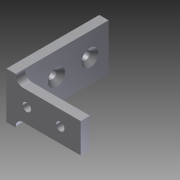
# Autodesk Inventor part: 13_0204_014
Saved by Autodesk Inventor 2012 SP1 (Build 160190100, 190)
## iProperties
Created: 2013-03-28
Part Number: 13_0204_014
Material: Default
Document SubType Name: Modeling
Designer: vogel
Density: 1 g/cm^3
Author: vogel
Autodesk Inventor part; units mm, degrees
ref_plane "YZ Plane" through (0, 0, 0) normal (1, 0, 0) x (0, 1, 0)
ref_plane "XZ Plane" through (0, 0, 0) normal (0, 1, 0) x (-1, 0, 0)
ref_plane "XY Plane" through (0, 0, 0) normal (0, 0, 1) x (1, 0, 0)
sketch "Skizze1" plane through (0, 0, 0) normal (0, 0, 1) x (1, 0, 0)
  line L0 (5, 5) -> (5, 50)
  line L1 (5, 50) -> (0, 50)
  line L2 (0, 50) -> (0, 0)
  line L3 (5, 5) -> (50, 5)
  line L4 (50, 5) -> (50, 0)
  line L5 (-10, 0) -> (60, 0) projected
  line L6 (0, -10) -> (0, 60) projected
  line L7 (0, 0) -> (50, 0)
  dimension "d3" = 5
  dimension "d4" = 5
  dimension "d5" = 50
  dimension "d6" = 50
  constraints: 12 end point, 2 collinear, 2 perpendicular, 1 horizontal, 1 parallel
  measures "d3" distance between parallel lines of L0 L2
  measures "d4" distance between parallel lines of L5 L3
  measures "d5" distance of L1.end L2.end
  measures "d6" distance of L2.end L4.end
extrude "Extrusion1" add sketch "Skizze1" along normal blind 25
sketch "Skizze3" plane through (0, 0, 0) normal (0, -1, 0) x (1, 0, 0)
  line L0 (0, 0) -> (0, 25) projected
  line L1 (50, 0) -> (0, 0) projected
  line L2 (50, 0) -> (50, 25) projected
  line L3 (50, 25) -> (40, 25)
  line L4 (40, 25) -> (40, 0)
  line L5 (40, 0) -> (50, 0)
  line L6 (50, 0) -> (50, 25)
  dimension "d9" = 40
  constraints: 8 end point, 2 parallel, 1 horizontal, 1 perpendicular, 1 point on line
  measures "d9" distance between parallel lines of L4 L0
extrude "Extrusion2" cut sketch "Skizze3" against normal through all
sketch "Skizze4" plane through (0, 0, 0) normal (0, -1, 0) x (1, 0, 0)
  line L0 (40, 0) -> (40, 25) projected
  line L1 (40, 25) -> (0, 25) projected
  line L2 (0, 0) -> (0, 25) projected
  line L3 (5, 0) -> (5, 25) projected
  line L4 (40, 25) -> (5, 25)
  line L5 (5, 25) -> (5, 20.5)
  line L6 (5, 20.5) -> (40, 20.5)
  line L7 (40, 20.5) -> (40, 25)
  line L8 (5, 0) -> (40, 0)
  line L9 (40, 0) -> (40, 4.5)
  line L10 (40, 4.5) -> (5, 4.5)
  line L11 (5, 4.5) -> (5, 0)
  line L12 (0, 12.5) -> (40, 12.5)
  dimension "d12" = 16
  constraints: 18 end point, 4 parallel, 2 horizontal, 2 midpoint, 2 perpendicular, 1 collinear, 1 point on line, 1 other
  measures "d12" distance between parallel lines of L10 L6
extrude "Extrusion3" cut sketch "Skizze4" against normal through all contours L8 L3 L10 L0 | L6 L3 L1 L0
sketch "Skizze5" plane through (0, 0, 0) normal (0, -1, 0) x (1, 0, 0)
  line L0 (40, 4.5) -> (40, 20.5) projected
  line L1 (0, 0) -> (0, 25) projected
  line L2 (0, 12.5) -> (40, 12.5)
  point P0 (11, 12.5)
  point P1 (29, 12.5)
  dimension "d15" = 18
  dimension "d16" = 11
  constraints: 2 end point, 2 midpoint, 2 point on line
  measures "d15" distance of point (29, 12.5) point (11, 12.5)
  measures "d16" distance from line of L1 point (11, 12.5)
hole "Bohrung1" at (11, 0, 12.5) at (29, 0, 12.5) direction (0, 1, 0) diameter 4.5 end through all
fillet "Rundung1" radius 4 2 edges at (5, 2.5, 20.5) (5, 2.5, 4.5)
sketch "Skizze6" plane through (5, 0, 0) normal (1, 0, 0) x (0, 0, -1)
  line L0 (0, 50) -> (-25, 50) projected
  line L1 (-0.5, 5) -> (-24.5, 5) projected
  line L2 (-12.5, 50) -> (-12.5, 10.6492)
  point P0 (-12.5, 40)
  point P1 (-12.5, 22)
  dimension "d25" = 10
  dimension "d26" = 18
  constraints: 2 end point, 2 point on line, 1 midpoint, 1 perpendicular
  measures "d25" distance from line of L0 point (-12.5, 40)
  measures "d26" distance of point (-12.5, 40) point (-12.5, 22)
hole "Bohrung2" at (5, 40, 12.5) at (5, 22, 12.5) direction (-1, 0, 0) diameter 4.5 end through all countersink diameter 9.2 countersink angle 90
